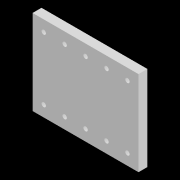
# Autodesk Inventor part: ArmServoMount
Saved by Autodesk Inventor 2020 (Build 240168000, 168)
## iProperties
Created: 2020-04-19
Part Number: ArmServoMount
Material: Generic
Document SubType Name: Sheet Metal
Designer: valer
Density: 1 g/cm^3
Sheet Metal Rule: Default
Appearance: Default
Author: valer
Autodesk Inventor part; units mm, degrees
ref_plane "YZ Plane" through (0, 0, 0) normal (1, 0, 0) x (0, 1, 0)
ref_plane "XZ Plane" through (0, 0, 0) normal (0, 1, 0) x (-1, 0, 0)
ref_plane "XY Plane" through (0, 0, 0) normal (0, 0, 1) x (1, 0, 0)
sketch "Sketch1" plane through (0, 0, 0) normal (0, 0, 1) x (1, 0, 0)
  circle A0 centre (48, 18) radius 1.25
  circle A1 centre (36, 18) radius 1.25
  circle A2 centre (24, 18) radius 1.25
  circle A3 centre (12, 18) radius 1.25
  circle A4 centre (0, 18) radius 1.25
  circle A5 centre (0, -18) radius 1.25
  circle A6 centre (12, -18) radius 1.25
  circle A7 centre (24, -18) radius 1.25
  circle A8 centre (36, -18) radius 1.25
  circle A9 centre (48, -18) radius 1.25
  line L0 (0, 18) -> (48, 18) construction
  line L1 (48, 18) -> (48, -18) construction
  line L2 (48, -18) -> (0, -18) construction
  line L3 (0, -18) -> (0, 18) construction
  line L4 (-6.35, 24.35) -> (54.35, 24.35)
  line L5 (54.35, 24.35) -> (54.35, -24.35)
  line L6 (54.35, -24.35) -> (-6.35, -24.35)
  line L7 (-6.35, -24.35) -> (-6.35, 24.35)
  point P0 (0, 0)
  point P1 (0, 0)
  dimension "d0" = 2.5
  dimension "d1" = 48
  dimension "d2" = 36
  dimension "d3" = 12
  dimension "d5" = 12
  dimension "d6" = 12
  dimension "d7" = 12
  dimension "d8" = 12
  dimension "d9" = 12
  dimension "d10" = 12
  dimension "d11" = 12
  dimension "d12" = 6.35
  dimension "d13" = 6.35
  dimension "d14" = 6.35
  dimension "d15" = 6.35
  measures "d0" diameter of A4
  measures "d1" distance between parallel lines of L1 L3
  measures "d2" distance of L2.end L0.start
  measures "d3" distance of L0.start A3.centre
  measures "d5" distance of A2.centre A3.centre
  measures "d6" distance of A1.centre A2.centre
  measures "d7" distance of A0.centre A1.centre
  measures "d8" distance of A6.centre A5.centre
  measures "d9" distance of A7.centre A6.centre
  measures "d10" distance of A8.centre A7.centre
  measures "d11" distance of L1.end A8.centre
  measures "d12" distance between parallel lines of L7 L3
  measures "d13" distance between parallel lines of L4 L0
  measures "d14" distance between parallel lines of L5 L1
  measures "d15" distance between parallel lines of L6 L2
extrude "Plate1" add sketch "Sketch1" along normal blind 5.08
equation "\"d16\" = Thickness"
equation "\"BendRadius\" = Thickness"
equation "\"BendReliefWidth\" = Thickness"
equation "\"BendReliefDepth\" = 0.5 * Thickness"
equation "\"CornerReliefSize\" = 4 * Thickness"
equation "\"MinimumRemnant\" = 2 * Thickness"
equation "\"TransitionRadius\" = BendRadius"
equation "\"JacobiRadiusSize\" = BendRadius"
equation "\"GapSize\" = Thickness"
equation "\"Thickness\" = 5.08"
body "Solid1"
